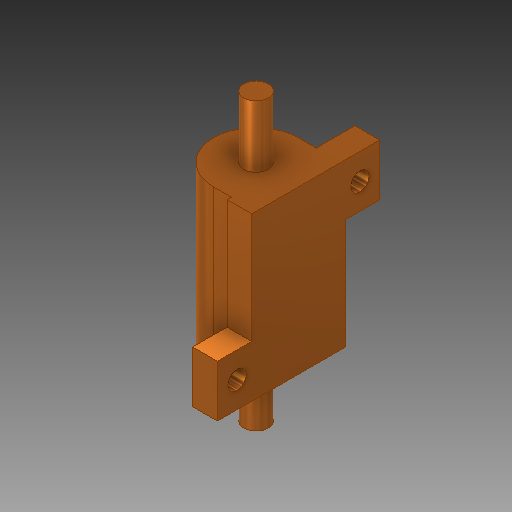
# Autodesk Inventor part: Power Resistor - HSA25
Saved by Autodesk Inventor 2017 (Build 210142000, 142)
## iProperties
Created: 2022-12-04
Part Number: Power Resistor - HSA25
Material: Gold
Document SubType Name: Modeling
Designer: Win240
Mass: 273.3 g
Surface Area: 53.5113 cm^2
Volume: 14.1606 cm^3
Density: 19.3 g/cm^3
Appearance: Metal 1600F Hot
Author: Win240
Autodesk Inventor part; units mm, degrees
ref_plane "YZ Plane" through (0, 0, 0) normal (1, 0, 0) x (0, 1, 0)
ref_plane "XZ Plane" through (0, 0, 0) normal (0, 1, 0) x (-1, 0, 0)
ref_plane "XY Plane" through (0, 0, 0) normal (0, 0, 1) x (1, 0, 0)
sketch "Sketch1" plane through (0, 0, 0) normal (0, 1, 0) x (-1, 0, 0)
  arc A0 (5.5, -5.5) -> (11, 0) centre (5.5, 0) ccw
  line L0 (3.2, -5.5) -> (3.2, -10.5)
  line L1 (3.2, -10.5) -> (0, -10.5)
  line L2 (0, -10.5) -> (0, 10.5)
  line L3 (0, 10.5) -> (3.2, 10.5)
  line L4 (3.2, 10.5) -> (3.2, 5.5)
  arc A1 (11, 0) -> (5.5, 5.5) centre (5.5, 0) ccw
  line L5 (3.2, 5.5) -> (11, 0) construction
  line L6 (3.2, -5.5) -> (11, 0) construction
  line L7 (5.5, 5.5) -> (3.2, 5.5)
  line L8 (3.2, -5.5) -> (5.5, -5.5)
  point P0 (0, 0)
  point P1 (0, 0)
  dimension "d0" = 3.2
  dimension "d1" = 21
  dimension "d6" = 11
  dimension "d21" = 11
  constraints: 18 end point, 4 horizontal, 4 point on circle, 3 equal length, 3 tangent, 3 vertical, 2 centre point, 1 coincident, 1 concentric, 1 midpoint
  measures "d0" distance of L0.end L1.end
  measures "d1" distance of L1.end L2.end
  measures "d6" distance from line of L5.end L2
  measures "d21" distance between parallel lines of L8 L7
extrude "Extrusion1" add sketch "Sketch1" along normal blind 21
sketch "Sketch2" plane through (0, 0, 10.5) normal (1, 0, 0) x (0, 0, -1)
  circle A0 centre (18.45, 17.65) radius 1.2
  circle A1 centre (2.55, 3.35) radius 1.2
  line L0 (18.45, 17.65) -> (18.45, 3.35) construction
  line L1 (18.45, 3.35) -> (2.55, 3.35) construction
  line L2 (21, 0) -> (21, 21) projected
  line L3 (0, 0) -> (0, 21) projected
  line L4 (18.45, 17.65) -> (21, 17.65) construction
  line L5 (18.45, 17.65) -> (21, 21) construction
  line L6 (0, 0) -> (2.55, 3.35) construction
  line L7 (2.55, 3.35) -> (0, 3.35) construction
  line L8 (21, 14.3) -> (16.55, 14.3)
  line L9 (16.55, 14.3) -> (16.55, 0)
  line L10 (16.55, 0) -> (21, 0)
  line L11 (0, 6.7) -> (4.45, 6.7)
  line L12 (4.45, 6.7) -> (4.45, 21)
  line L13 (4.45, 21) -> (0, 21)
  line L14 (21, 14.3) -> (18.45, 17.65) construction
  point P0 (10.5, 0)
  dimension "d9" = 15.9
  dimension "d10" = 14.3
  dimension "d11" = 2.4
  dimension "d12" = 1.9
  constraints: 26 end point, 7 horizontal, 5 equal length, 4 point on line, 3 vertical, 2 centre point, 1 equal radius
  measures "d9" distance of L0.end L1.end
  measures "d10" distance of L0.start L0.end
  measures "d11" diameter of A0
  measures "d12" distance from line of L0.start L9
extrude "Extrusion2" cut sketch "Sketch2" against normal up to surface (3.2 mm away)
sketch "Sketch3" plane through (0, 0, 0) normal (0, -1, 0) x (1, 0, 0)
  arc A0 (-3.2, 5.5) -> (-3.2, -5.5) centre (-5.5, 0) ccw projected
  circle A1 centre (-5.5, 0) radius 1.5875
  point P0 (0, 0)
  dimension "d15" = 3.175
  constraints: 1 centre point, 1 coincident, 1 other
  measures "d15" diameter of A1
extrude "Extrusion3" add sketch "Sketch3" along normal blind 8
sketch "Sketch4" plane through (0, 21, 0) normal (0, 1, 0) x (1, 0, 0)
  arc A0 (-3.2, 5.5) -> (-3.2, -5.5) centre (-5.5, 0) ccw construction
  circle A1 centre (-5.5, 0) radius 1.5875
  point P0 (0, 0)
  dimension "d18" = 3.175
  constraints: 1 centre point, 1 coincident, 1 other
  measures "d18" diameter of A1
extrude "Extrusion4" add sketch "Sketch4" along normal blind 8
body "Solid1"
